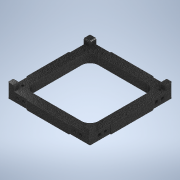
# Autodesk Inventor part: BottomSide
Saved by Autodesk Inventor 2022 (Build 260153000, 153)
## iProperties
Created: 2022-01-14
Part Number: BottomSide
Material: ABS Plastic
Document SubType Name: Modeling
Designer: Sergey
Density: 1.06 g/cm^3
Appearance: Black Cast
Author: Sergey
Autodesk Inventor part; units mm, degrees
ref_plane "YZ Plane" through (0, 0, 0) normal (1, 0, 0) x (0, 1, 0)
ref_plane "XZ Plane" through (0, 0, 0) normal (0, 1, 0) x (-1, 0, 0)
ref_plane "XY Plane" through (0, 0, 0) normal (0, 0, 1) x (1, 0, 0)
sketch "Sketch1" plane through (0, 0, 0) normal (0, 1, 0) x (-1, 0, 0)
  circle A0 centre (0, 0) radius 1.45
  circle A1 centre (0, -73.66) radius 1.45
  circle A2 centre (-85.73, -77.47) radius 1.45
  circle A3 centre (-85.73, 2.54) radius 1.45
  line L0 (7.135, 12.535) -> (-92.865, 12.535)
  line L1 (-92.865, 12.535) -> (-92.865, -87.465)
  line L2 (-92.865, -87.465) -> (7.135, -87.465)
  line L3 (7.135, -87.465) -> (7.135, 12.535)
  line L4 (0, 0) -> (7.135, 0)
  line L5 (-85.73, 2.54) -> (-92.865, 2.54)
  line L6 (-85.73, -77.47) -> (-85.73, -87.465)
  line L7 (-85.73, 2.54) -> (-85.73, 12.535)
  point P0 (0, 0)
  dimension "d0" = 73.66
  dimension "d1" = 80.01
  dimension "d2" = 85.73
  dimension "d3" = 2.54
  dimension "d4" = 3.81
  dimension "d6" = 2.9
  dimension "d7" = 100
  dimension "d8" = 100
  constraints: 16 end point, 5 point on line, 4 centre point, 4 perpendicular, 3 equal radius, 2 coincident, 2 equal length, 2 parallel, 1 horizontal, 1 vertical alignment
  measures "d0" distance of A1.centre point (0, 0)
  measures "d1" distance of L6.start L5.start
  measures "d2" horizontal distance of L5.start point (0, 0)
  measures "d3" vertical distance of L5.start point (0, 0)
  measures "d4" vertical distance of L6.start A1.centre
  measures "d6" diameter of A3
  measures "d7" distance of L2.end L1.end
  measures "d8" distance of L1.end L0.end
extrude "Extrusion1" add sketch "Sketch1" along normal blind 10 contours L3 L2 L1 L5 A3 L7 L0 | L7 A3 L5 L1 L0
sketch "Sketch4" plane through (0, 0, 0) normal (0, -1, 0) x (1, 0, 0)
  line L0 (92.865, -87.465) -> (-7.135, -87.465) projected
  line L1 (92.865, 12.535) -> (92.865, -87.465) projected
  line L2 (-7.135, 12.535) -> (92.865, 12.535) projected
  line L3 (-7.135, -87.465) -> (-7.135, 12.535) projected
  circle A0 centre (85.73, 2.54) radius 1.45 projected
  circle A1 centre (0, 0) radius 1.45 projected
  circle A2 centre (85.73, -77.47) radius 1.45 projected
  circle A3 centre (0, -73.66) radius 1.45 projected
  circle A4 centre (0, 0) radius 2.25
  circle A5 centre (0, -73.66) radius 2.25
  circle A6 centre (85.73, -77.47) radius 2.25
  circle A7 centre (85.73, 2.54) radius 2.25
  point P0 (0, 0)
  dimension "d13" = 4.5
  dimension "d14" = 4.5
  dimension "d15" = 4.5
  dimension "d16" = 4.5
  constraints: 4 centre point, 4 coincident
  measures "d13" diameter of A4
  measures "d14" diameter of A5
  measures "d15" diameter of A6
  measures "d16" diameter of A7
extrude "Extrusion2" cut sketch "Sketch4" against normal blind 6.2 contours A0 | A1 | A2 | A3 | A4 | A5 | A6 | A7
sketch "Sketch5" plane through (0, 0, 0) normal (0, -1, 0) x (1, 0, 0)
  circle A0 centre (85.73, 2.54) radius 2.25 projected
  circle A1 centre (0, 0) radius 2.25 projected
  circle A2 centre (85.73, -77.47) radius 2.25 projected
  circle A3 centre (0, -73.66) radius 2.25 projected
  line L0 (92.865, -87.465) -> (-7.135, -87.465) projected
  line L1 (92.865, 12.535) -> (92.865, -87.465) projected
  line L2 (-7.135, 12.535) -> (92.865, 12.535) projected
  line L3 (-7.135, -87.465) -> (-7.135, 12.535) projected
  line L4 (-7.135, -87.465) -> (92.865, 12.535)
  line L5 (-7.135, -12.465) -> (-5.935, -12.465)
  line L6 (-5.935, -12.465) -> (-5.935, 11.335)
  line L7 (-5.935, 11.335) -> (17.865, 11.335)
  line L8 (17.865, 11.335) -> (17.865, 12.535)
  line L9 (-7.135, 12.535) -> (92.865, 12.535) projected
  line L10 (17.865, -86.265) -> (-5.935, -86.265)
  line L11 (-5.935, -62.465) -> (-7.135, -62.465)
  line L12 (-5.935, -86.265) -> (-5.935, -62.465)
  line L13 (17.865, -87.465) -> (17.865, -86.265)
  line L14 (91.665, -62.465) -> (91.665, -86.265)
  line L15 (67.865, -86.265) -> (67.865, -87.465)
  line L16 (91.665, -86.265) -> (67.865, -86.265)
  line L17 (92.865, -62.465) -> (91.665, -62.465)
  line L18 (67.865, 11.335) -> (91.665, 11.335)
  line L19 (91.665, -12.465) -> (92.865, -12.465)
  line L20 (91.665, 11.335) -> (91.665, -12.465)
  line L21 (67.865, 12.535) -> (67.865, 11.335)
  point P0 (0, 0)
  point P1 (42.865, -37.465)
  point P2 (17.865, 12.535)
  point P3 (17.865, -87.465)
  point P4 (-7.135, -62.465)
  point P5 (67.865, -87.465)
  point P6 (92.865, -62.465)
  point P7 (67.865, 12.535)
  point P8 (92.865, -12.465)
  dimension "d19" = 1.2
  dimension "d20" = 1.2
  dimension "d21" = 25
  dimension "d22" = 25
  dimension "d27" = 360
  constraints: 34 end point, 3 perpendicular, 2 point on line, 1 horizontal, 1 midpoint, 37 other
  measures "d19" distance of L5.start L5.end
  measures "d20" distance of L7.end L8.end
  measures "d21" distance between parallel lines of L2 L5
  measures "d22" distance between parallel lines of L8 L3
extrude "Extrusion3" cut sketch "Sketch5" along normal through all both and the other way through all contours L18 L21 L2 L4 | L4 L1 L19 L20 | L10 L13 L0 L4 | L4 L3 L11 L12 | L1 L0 L15 L16 L14 L17 | L8 L7 L6 L5 L3 L2
fillet "Fillet1" radius 1 4 edges at (-5.935, 5, -86.265) (91.665, 5, -86.265) (-5.935, 5, 11.335) (91.665, 5, 11.335)
sketch "Sketch6" plane through (0, 10, 0) normal (0, 1, 0) x (1, 0, 0)
  arc A0 (90.665, -11.335) -> (91.665, -10.335) centre (90.665, -10.335) ccw projected
  line L0 (91.665, -10.335) -> (91.665, 12.465) projected
  line L1 (91.665, 12.465) -> (92.865, 12.465) projected
  line L2 (92.865, 12.465) -> (92.865, 62.465) projected
  line L3 (92.865, 62.465) -> (91.665, 62.465) projected
  line L4 (91.665, 62.465) -> (91.665, 85.265) projected
  arc A1 (91.665, 85.265) -> (90.665, 86.265) centre (90.665, 85.265) ccw projected
  line L5 (90.665, 86.265) -> (67.865, 86.265) projected
  line L6 (67.865, 86.265) -> (67.865, 87.465) projected
  line L7 (67.865, 87.465) -> (17.865, 87.465) projected
  line L8 (17.865, 87.465) -> (17.865, 86.265) projected
  line L9 (17.865, 86.265) -> (-4.935, 86.265) projected
  arc A2 (-4.935, 86.265) -> (-5.935, 85.265) centre (-4.935, 85.265) ccw projected
  line L10 (-5.935, 85.265) -> (-5.935, 62.465) projected
  line L11 (-5.935, 62.465) -> (-7.135, 62.465) projected
  line L12 (-7.135, 62.465) -> (-7.135, 12.465) projected
  line L13 (-7.135, 12.465) -> (-5.935, 12.465) projected
  line L14 (-5.935, 12.465) -> (-5.935, -10.335) projected
  arc A3 (-5.935, -10.335) -> (-4.935, -11.335) centre (-4.935, -10.335) ccw projected
  line L15 (-4.935, -11.335) -> (17.865, -11.335) projected
  line L16 (17.865, -11.335) -> (17.865, -12.535) projected
  line L17 (17.865, -12.535) -> (67.865, -12.535) projected
  line L18 (67.865, -12.535) -> (67.865, -11.335) projected
  line L19 (67.865, -11.335) -> (90.665, -11.335) projected
  circle A4 centre (0, 73.66) radius 1.45 projected
  circle A5 centre (85.73, 77.47) radius 1.45 projected
  circle A6 centre (0, 0) radius 1.45 projected
  circle A7 centre (85.73, -2.54) radius 1.45 projected
  line L20 (-5.935, -11.335) -> (1.365, -11.335)
  line L21 (1.365, -11.335) -> (1.365, -4.035)
  line L22 (1.365, -4.035) -> (-5.935, -4.035)
  line L23 (-5.935, -4.035) -> (-5.935, -11.335)
  line L24 (-7.135, 62.465) -> (-7.135, 12.465) projected
  line L25 (-7.135, 37.465) -> (92.865, 37.465)
  line L26 (92.865, 12.465) -> (92.865, 62.465) projected
  line L27 (84.365, -11.335) -> (91.665, -11.335)
  line L28 (84.365, -4.035) -> (84.365, -11.335)
  line L29 (91.665, -4.035) -> (84.365, -4.035)
  line L30 (91.665, -11.335) -> (91.665, -4.035)
  line L31 (91.665, 78.965) -> (91.665, 86.265)
  line L32 (84.365, 78.965) -> (91.665, 78.965)
  line L33 (84.365, 86.265) -> (84.365, 78.965)
  line L34 (91.665, 86.265) -> (84.365, 86.265)
  line L35 (1.365, 86.265) -> (-5.935, 86.265)
  line L36 (1.365, 78.965) -> (1.365, 86.265)
  line L37 (-5.935, 78.965) -> (1.365, 78.965)
  line L38 (-5.935, 86.265) -> (-5.935, 78.965)
  point P0 (0, 0)
  point P1 (-5.935, -4.035)
  point P2 (1.365, -11.335)
  point P3 (42.865, 37.465)
  point P4 (-5.935, 78.965)
  point P5 (84.365, 86.265)
  point P6 (85.6076, 78.965)
  point P7 (85.8524, 78.965)
  point P8 (91.665, 78.965)
  point P9 (91.665, -4.035)
  point P10 (84.365, -11.335)
  dimension "d30" = 7.3
  dimension "d31" = 7.3
  dimension "d39" = 360
  constraints: 34 end point, 3 midpoint, 2 parallel, 1 horizontal, 1 perpendicular, 33 other
  measures "d30" distance of L22.end L21.end
  measures "d31" distance of L21.end L20.end
extrude "Extrusion4" add sketch "Sketch6" along normal blind 6.5 contours L19 L28 L29 L0 A0 | L15 A3 L14 L22 L21 | L32 L33 L5 A1 L4 | L10 A2 L9 L36 L37
chamfer "Chamfer1" distance 1 angle 45 12 edges at (-2.285, 16.5, 4.035) (1.365, 16.5, 7.685) (1.365, 16.5, -82.615) (-2.285, 16.5, -78.965) (84.365, 16.5, -82.615) (88.015, 16.5, -78.965) (88.015, 16.5, 4.035) (84.365, 16.5, 7.685) (84.365, 13.25, 4.035) (1.365, 13.25, 4.035) (84.365, 13.25, -78.965) (1.365, 13.25, -78.965)
sketch "Sketch7" plane through (0, 10, 0) normal (0, 1, 0) x (1, 0, 0)
  circle A0 centre (85.73, -2.54) radius 1.45 projected
  circle A1 centre (0, 0) radius 1.45 projected
  circle A2 centre (85.73, 77.47) radius 1.45 projected
  circle A3 centre (0, 73.66) radius 1.45 projected
  line L0 (1.365, 86.265) -> (1.365, 79.965) projected
  line L1 (0.365, 78.965) -> (-5.935, 78.965) projected
  line L2 (-5.935, 78.965) -> (-5.935, 62.465) projected
  line L3 (-5.935, 62.465) -> (-7.135, 62.465) projected
  line L4 (-7.135, 62.465) -> (-7.135, 12.465) projected
  line L5 (-7.135, 12.465) -> (-5.935, 12.465) projected
  line L6 (-5.935, 12.465) -> (-5.935, -4.035) projected
  line L7 (-5.935, -4.035) -> (0.365, -4.035) projected
  line L8 (1.365, -5.035) -> (1.365, -11.335) projected
  line L9 (1.365, -11.335) -> (17.865, -11.335) projected
  line L10 (17.865, -11.335) -> (17.865, -12.535) projected
  line L11 (17.865, -12.535) -> (67.865, -12.535) projected
  line L12 (67.865, -12.535) -> (67.865, -11.335) projected
  line L13 (67.865, -11.335) -> (84.365, -11.335) projected
  line L14 (84.365, -11.335) -> (84.365, -5.035) projected
  line L15 (85.365, -4.035) -> (91.665, -4.035) projected
  line L16 (91.665, -4.035) -> (91.665, 12.465) projected
  line L17 (91.665, 12.465) -> (92.865, 12.465) projected
  line L18 (92.865, 12.465) -> (92.865, 62.465) projected
  line L19 (92.865, 62.465) -> (91.665, 62.465) projected
  line L20 (91.665, 62.465) -> (91.665, 78.965) projected
  line L21 (91.665, 78.965) -> (85.365, 78.965) projected
  line L22 (84.365, 79.965) -> (84.365, 86.265) projected
  line L23 (84.365, 86.265) -> (67.865, 86.265) projected
  line L24 (67.865, 86.265) -> (67.865, 87.465) projected
  line L25 (67.865, 87.465) -> (17.865, 87.465) projected
  line L26 (17.865, 87.465) -> (17.865, 86.265) projected
  line L27 (17.865, 86.265) -> (1.365, 86.265) projected
  line L28 (3.865, 76.465) -> (81.865, 76.465)
  line L29 (81.865, 76.465) -> (81.865, -1.535)
  line L30 (81.865, -1.535) -> (3.865, -1.535)
  line L31 (3.865, -1.535) -> (3.865, 76.465)
  line L32 (0.365, 78.965) -> (1.365, 79.965) projected
  line L33 (1.365, -5.035) -> (0.365, -4.035) projected
  line L34 (85.365, -4.035) -> (84.365, -5.035) projected
  line L35 (84.365, 79.965) -> (85.365, 78.965) projected
  point P0 (0, 0)
  dimension "d50" = 11
  dimension "d51" = 11
  dimension "d52" = 11
  dimension "d53" = 11
  constraints: 8 end point, 2 parallel, 1 horizontal, 1 perpendicular
  measures "d50" distance between parallel lines of L31 L4
  measures "d51" distance between parallel lines of L18 L29
  measures "d52" distance between parallel lines of L25 L28
  measures "d53" distance between parallel lines of L11 L30
extrude "Extrusion5" cut sketch "Sketch7" against normal blind 10 contours L28 L29 L30 L31
fillet "Fillet2" radius 10 4 edges at (3.865, 5, -76.465) (81.865, 5, -76.465) (81.865, 5, 1.535) (3.865, 5, 1.535)
sketch "Sketch8" plane through (92.865, 0, -12.465) normal (1, 0, 0) x (0, 0, -1)
  line L0 (-25, 5) -> (75, 5)
  circle A0 centre (-5.5, 5) radius 2.1
  circle A1 centre (55.5, 5) radius 2.1
  line L1 (0, 0) -> (50, 0) projected
  line L2 (0, 10) -> (50, 10) projected
  circle A2 centre (62.5, 5) radius 2.1
  line L3 (75, 10) -> (75, 0) projected
  circle A3 centre (-12.5, 5) radius 2.1
  point P0 (-12.465, 0)
  point P1 (25, 5)
  dimension "d57" = 30.5
  dimension "d58" = 30.5
  dimension "d59" = 4.2
  dimension "d60" = 4.2
  dimension "d75" = 5
  dimension "d80" = 4.2
  dimension "d81" = 19.5
  dimension "d82" = 7
  dimension "d83" = 4.2
  dimension "d84" = 7
  constraints: 4 centre point, 4 point on line, 2 end point, 1 midpoint
  measures "d57" distance of point (25, 5) A0.centre
  measures "d58" distance of point (25, 5) A1.centre
  measures "d59" diameter of A0
  measures "d60" diameter of A1
  measures "d75" distance between parallel lines of L2 L0
  measures "d80" diameter of A2
  measures "d81" distance from line of L3 A1.centre
  measures "d82" distance of A2.centre A1.centre
  measures "d83" diameter of A3
  measures "d84" distance of A0.centre A3.centre
extrude "Extrusion6" cut sketch "Sketch8" against normal blind 7.7
sketch "Sketch9" plane through (67.865, 0, -86.265) normal (0, 0, -1) x (-1, 0, 0)
  line L0 (-25, 10) -> (-25, 0) projected
  circle A0 centre (-5.5, 5) radius 2.1
  circle A1 centre (55.5, 5) radius 2.1
  line L1 (-16.5, 10) -> (0, 10) projected
  line L2 (50, 10) -> (66.5, 10) projected
  line L3 (75, 10) -> (75, 0) projected
  circle A2 centre (62.5, 5) radius 2.1
  circle A3 centre (-12.5, 5) radius 2.1
  point P0 (67.865, 0)
  dimension "d63" = 4.2
  dimension "d64" = 4.2
  dimension "d76" = 5
  dimension "d77" = 5
  dimension "d78" = 19.5
  dimension "d79" = 19.5
  dimension "d85" = 4.2
  dimension "d86" = 4.2
  dimension "d87" = 7
  dimension "d88" = 7
  constraints: 4 centre point
  measures "d63" diameter of A0
  measures "d64" diameter of A1
  measures "d76" distance from line of A0.centre L1
  measures "d77" distance from line of A1.centre L2
  measures "d78" distance from line of L3 A1.centre
  measures "d79" distance from line of L0 A0.centre
  measures "d85" diameter of A2
  measures "d86" diameter of A3
  measures "d87" distance of A0.centre A3.centre
  measures "d88" distance of A1.centre A2.centre
extrude "Extrusion7" cut sketch "Sketch9" against normal blind 6.5
sketch "Sketch10" plane through (-7.135, 0, -62.465) normal (-1, 0, 0) x (0, 0, 1)
  line L0 (-25, 0) -> (-25, 10) projected
  line L1 (75, 10) -> (75, 0) projected
  line L2 (-25, 5) -> (75, 5)
  circle A0 centre (-5.5, 5) radius 2.1 projected
  circle A1 centre (-5.5, 5) radius 2.1
  circle A2 centre (55.5, 5) radius 2.1 projected
  circle A3 centre (55.5, 5) radius 2.1
  circle A4 centre (-12.5, 5) radius 2.1
  circle A5 centre (62.5, 5) radius 2.1 projected
  circle A6 centre (62.5, 5) radius 2.1
  point P0 (62.465, 0)
  point P1 (25, 5)
  dimension "d69" = 4.2
  dimension "d89" = 4.2
  dimension "d90" = 7
  constraints: 4 centre point, 3 coincident, 3 midpoint, 2 end point, 1 point on line
  measures "d69" diameter of A1
  measures "d89" diameter of A4
  measures "d90" distance of A1.centre A4.centre
extrude "Extrusion8" cut sketch "Sketch10" against normal blind 7.7
sketch "Sketch11" plane through (17.865, 0, 11.335) normal (0, 0, 1) x (1, 0, 0)
  line L0 (-25, 0) -> (-25, 10) projected
  line L1 (75, 10) -> (75, 0) projected
  line L2 (-25, 5) -> (75, 5)
  circle A0 centre (-5.5, 5) radius 2.1 projected
  circle A1 centre (-5.5, 5) radius 2.1
  circle A2 centre (55.5, 5) radius 2.1 projected
  circle A3 centre (55.5, 5) radius 2.1
  circle A4 centre (-12.5, 5) radius 2.1
  circle A5 centre (62.5, 5) radius 2.1 projected
  circle A6 centre (62.5, 5) radius 2.1
  point P0 (-17.865, 0)
  dimension "d91" = 4.2
  dimension "d92" = 4.2
  dimension "d93" = 7
  dimension "d94" = 19.5
  constraints: 4 centre point, 3 coincident, 2 end point, 2 midpoint, 1 point on line
  measures "d91" diameter of A4
  measures "d92" diameter of A6
  measures "d93" distance of A1.centre A4.centre
  measures "d94" distance from line of L0 A1.centre
extrude "Extrusion9" cut sketch "Sketch11" against normal blind 6.5
body "Solid1"
